# Autodesk Inventor part: AIN6-7_1X02_NO_SILK
Saved by Autodesk Inventor 2016 (Build 200138000, 138)
## iProperties
Created: 2016-04-08
Part Number: AIN6-7_1X02_NO_SILK
Material: Generic
Document SubType Name: Modeling
Designer: Paschalis
Density: 1 g/cm^3
Appearance: 1X02_NO_SILK, AIN6-7_1X02_NO_SILK
Author: Paschalis
Autodesk Inventor part; units mm, degrees
ref_plane "YZ Plane" through (0, 0, 0) normal (1, 0, 0) x (0, 1, 0)
ref_plane "XZ Plane" through (0, 0, 0) normal (0, 1, 0) x (-1, 0, 0)
ref_plane "XY Plane" through (0, 0, 0) normal (0, 0, 1) x (1, 0, 0)
sketch "1X02_NO_SILK, AIN6-7_1X02_NO_SILK_9" plane through (0, 0, 0) normal (0, 0, 1) x (1, 0, 0)
  line L0 (-0.254, 0.254) -> (2.794, 0.254)
  line L1 (2.794, 0.254) -> (2.794, -0.254)
  line L2 (2.794, -0.254) -> (-0.254, -0.254)
  line L3 (-0.254, -0.254) -> (-0.254, 0.254)
  constraints: 8 end point
extrude "Extrusion1" add sketch "1X02_NO_SILK, AIN6-7_1X02_NO_SILK_9" along normal blind 1
body "Solid1"
